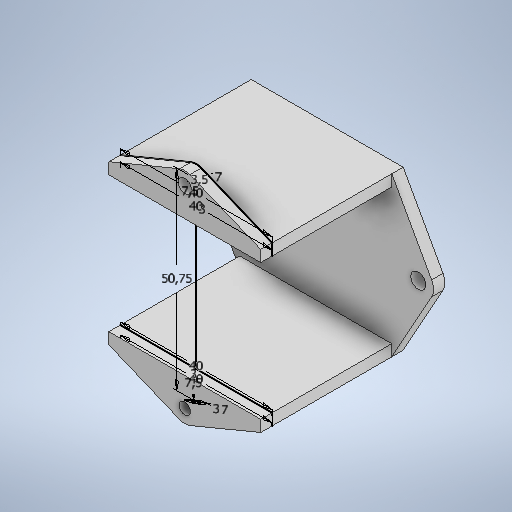
# Autodesk Inventor part: Mount
Saved by Autodesk Inventor 2025.2 (Build 292293000, 293)
## iProperties
Created: 2025-05-29
Part Number: Mount
Material: Generic
Document SubType Name: Modeling
Designer: Simon
Density: 1 g/cm^3
Appearance: Default
Author: Simon
Autodesk Inventor part; units mm, degrees
ref_plane "YZ Plane" through (0, 0, 0) normal (1, 0, 0) x (0, 1, 0)
ref_plane "XZ Plane" through (0, 0, 0) normal (0, 1, 0) x (-1, 0, 0)
ref_plane "XY Plane" through (0, 0, 0) normal (0, 0, 1) x (1, 0, 0)
sketch "Sketch1" plane through (0, 0, 0) normal (0, 0, 1) x (1, 0, 0)
  circle A0 centre (0, 0) radius 1.75
  line L0 (0, 0) -> (0, -50.75)
  circle A1 centre (0, -50.75) radius 1.5
  line L1 (0, 0) -> (0, -7.5)
  line L2 (0, -7.5) -> (0, -4.5)
  line L3 (-20, -7.5) -> (20, -7.5)
  line L4 (-20, -4.5) -> (20, -4.5)
  circle A2 centre (0, 0) radius 3.5
  line L5 (-20, -4.5) -> (-1.34, 3.2333)
  line L6 (20, -4.5) -> (1.34, 3.2333)
  line L7 (-20, -4.5) -> (-20, -7.5)
  line L8 (20, -4.5) -> (20, -7.5)
  line L9 (0, -50.75) -> (0, -43.25)
  line L10 (0, -43.25) -> (0, -46.25)
  line L11 (-20, -43.25) -> (20, -43.25)
  line L12 (-20, -46.25) -> (20, -46.25)
  circle A3 centre (0, -50.75) radius 3.5
  line L13 (-20, -43.25) -> (-20, -46.25)
  line L14 (-20, -46.25) -> (-1.34, -53.9833)
  line L15 (20, -43.25) -> (20, -46.25)
  line L16 (20, -46.25) -> (1.34, -53.9833)
  dimension "d0" = 3.5
  dimension "d1" = 50.75
  dimension "d2" = 3
  dimension "d3" = 7.5
  dimension "d4" = 3
  dimension "d5" = 40
  dimension "d6" = 40
  dimension "d7" = 7
  dimension "d8" = 7.5
  dimension "d9" = 3
  dimension "d10" = 40
  dimension "d11" = 40
  dimension "d12" = 7
  constraints: 34 end point, 4 centre point, 4 coincident, 4 midpoint, 4 point on circle, 4 point on line, 4 tangent, 3 horizontal, 1 parallel, 1 vertical
  measures "d0" diameter of A0
  measures "d1" distance of L0.start L0.end
  measures "d2" diameter of A1
  measures "d3" distance of L0.start L1.end
  measures "d4" distance of L1.end L2.end
  measures "d5" distance of L3.start L3.end
  measures "d6" distance of L4.start L4.end
  measures "d7" diameter of A2
  measures "d8" distance of L9.start L9.end
  measures "d9" distance of L9.end L10.end
  measures "d10" distance of L11.start L11.end
  measures "d11" distance of L12.start L12.end
  measures "d12" diameter of A3
extrude "Extrusion1" add sketch "Sketch1" along normal blind 3
extrude "Extrusion2" add sketch "Sketch1" against normal blind 31.5 contours L4 L8 L3 L0 | L0 L3 L7 L4 | L11 L15 L12 L0 | L0 L12 L13 L11
sketch "Sketch2" plane through (0, 0, -31.5) normal (0, 0, -1) x (-1, 0, 0)
  line L0 (-20, -7.5) -> (-20, -4.5) projected
  line L1 (-20, -4.5) -> (20, -4.5)
  line L2 (20, -4.5) -> (20, -46.25)
  line L3 (20, -46.25) -> (-20, -46.25)
  line L4 (-20, -46.25) -> (-20, -4.5)
  line L5 (20, -7.5) -> (-20, -7.5) projected
  line L6 (0, -7.5) -> (0, -25.375)
  line L7 (-20, -43.25) -> (20, -43.25) projected
  line L8 (-27, -25.375) -> (27, -25.375)
  circle A0 centre (-27, -25.375) radius 4
  circle A1 centre (-27, -25.375) radius 2
  circle A2 centre (27, -25.375) radius 4
  circle A3 centre (27, -25.375) radius 2
  line L9 (-20, -4.5) -> (-30.4983, -23.4354)
  line L10 (-1.34, -53.9833) -> (-20, -46.25) projected
  line L11 (-20, -46.25) -> (-30.4983, -27.3146)
  line L12 (20, -46.25) -> (30.4983, -27.3146)
  line L13 (20, -4.5) -> (30.4983, -23.4354)
  point P0 (0, 0)
  dimension "d17" = 17.875
  dimension "d18" = 54
  dimension "d19" = 8
  dimension "d20" = 4
  dimension "d21" = 8
  dimension "d22" = 4
  constraints: 20 end point, 4 centre point, 4 coincident, 4 point on circle, 4 tangent, 3 perpendicular, 2 midpoint, 2 parallel, 1 horizontal
  measures "d17" distance of L6.start L6.end
  measures "d18" distance of L8.start L8.end
  measures "d19" diameter of A0
  measures "d20" diameter of A1
  measures "d21" diameter of A2
  measures "d22" diameter of A3
extrude "Extrusion3" add sketch "Sketch2" along normal blind 3
body "Solid1"
